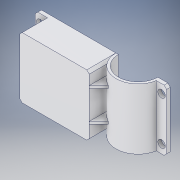
# Autodesk Inventor part: KS  Dianteiro Front
Saved by Autodesk Inventor 2019 (Build 230136000, 136)
## iProperties
Created: 2021-05-20
Part Number: KS  Dianteiro Front
Material: Genérico
Document SubType Name: Modeling
Designer: lukas
Density: 1 g/cm^3
Appearance: PTFE
Author: lukas
Autodesk Inventor part; units mm, degrees
ref_plane "YZ Plane" through (0, 0, 0) normal (1, 0, 0) x (0, 1, 0)
ref_plane "XZ Plane" through (0, 0, 0) normal (0, 1, 0) x (-1, 0, 0)
ref_plane "XY Plane" through (0, 0, 0) normal (0, 0, 1) x (1, 0, 0)
sketch "Esboço1" plane through (0, 0, 0) normal (0, 1, 0) x (-1, 0, 0)
  line L0 (-28, -11.75) -> (28, -11.75)
  line L1 (28, -11.75) -> (28, 11.75)
  line L2 (28, 11.75) -> (-28, 11.75)
  line L3 (-28, 11.75) -> (-28, -11.75)
  line L4 (-28, -11.75) -> (28, 11.75) construction
  line L5 (28, -11.75) -> (-28, 11.75) construction
  point P0 (0, 0)
  dimension "d0" = 56
  dimension "d1" = 23.5
  constraints: 12 end point, 2 midpoint, 2 parallel, 1 horizontal, 1 perpendicular
  measures "d0" distance of L2.end L1.end
  measures "d1" distance of L1.end L0.end
extrude "Extrusão1" add sketch "Esboço1" along normal blind 49
sketch "Esboço2" plane through (28, 0, -11.75) normal (0, 0, -1) x (-1, 0, 0)
  line L0 (0, 49) -> (56, 49) projected
  line L1 (0, 49) -> (-33.75, 49)
  line L2 (-33.75, 49) -> (-33.75, 0)
  line L3 (0, 0) -> (56, 0) projected
  line L4 (-33.75, 0) -> (0, 0)
  line L5 (0, 0) -> (0, 49)
  point P0 (28, 0)
  dimension "d4" = 33.75
  constraints: 8 end point, 3 perpendicular, 1 horizontal
  measures "d4" distance of L0.start L1.end
extrude "Extrusão2" add sketch "Esboço2" against normal blind 17.875
sketch "Esboço3" plane through (0, 49, 0) normal (0, 1, 0) x (1, 0, 0)
  line L0 (-28, 11.75) -> (61.75, 11.75) projected
  line L1 (61.75, 11.75) -> (59.75, 11.75)
  line L2 (59.75, 11.75) -> (43.875, 11.75)
  circle A0 centre (43.875, 11.75) radius 15.875
  point P0 (0, 0)
  dimension "d7" = 2
  dimension "d8" = 15.875
  constraints: 4 end point, 2 point on line, 1 coincident, 1 horizontal alignment, 2 other
  measures "d7" distance of L0.end L1.end
  measures "d8" distance of L1.end L2.end
extrude "Extrusão3" cut sketch "Esboço3" against normal blind 49
sketch "Esboço4" plane through (61.75, 0, -11.75) normal (0, 0, -1) x (-1, 0, 0)
  line L0 (0, 49) -> (33.75, 49) projected
  line L1 (33.75, 0) -> (0, 0) projected
  line L2 (0, 49) -> (0, 0)
  line L3 (0, 0) -> (-8, 0)
  line L4 (-8, 0) -> (-8, 49)
  line L5 (-8, 49) -> (0, 49)
  line L6 (-4, 0) -> (-4, 7)
  line L7 (-4, 49) -> (-4, 42)
  circle A0 centre (-4, 42) radius 3
  circle A1 centre (-4, 7) radius 3
  point P0 (61.75, 0)
  dimension "d11" = 8
  dimension "d12" = 7
  dimension "d13" = 7
  dimension "d14" = 6
  dimension "d15" = 6
  constraints: 12 end point, 3 vertical, 2 centre point, 2 coincident, 2 midpoint, 2 perpendicular, 1 horizontal
  measures "d11" distance of L1.end L3.end
  measures "d12" distance of L6.start L6.end
  measures "d13" distance of L7.start L7.end
  measures "d14" diameter of A0
  measures "d15" diameter of A1
extrude "Extrusão4" add sketch "Esboço4" against normal blind 3
sketch "Esboço5" plane through (0, 49, 0) normal (0, 1, 0) x (1, 0, 0)
  arc A0 (28, 11.75) -> (59.75, 11.75) centre (43.875, 11.75) ccw projected
  circle A1 centre (43.875, 11.75) radius 17.875
  line L0 (61.75, -6.125) -> (28, -6.125) projected
  line L1 (69.75, 8.75) -> (61.75, 8.75) projected
  line L2 (61.75, 8.75) -> (61.4965, 8.75)
  line L3 (61.75, 8.75) -> (61.75, -6.125)
  line L4 (43.875, -6.125) -> (61.75, -6.125)
  line L5 (28, -11.75) -> (28, -6.125) projected
  line L6 (43.875, -6.125) -> (28, -6.125)
  line L7 (28, -6.125) -> (28, 3.5342)
  point P0 (0, 0)
  constraints: 10 end point, 3 perpendicular, 3 point on circle, 2 tangent, 1 centre point, 1 coincident, 1 collinear, 1 horizontal, 1 point on line
extrude "Extrusão5" cut sketch "Esboço5" against normal blind 49 contours A1 L0 L7 | L2 L3 L0 A1
sketch "Esboço6" plane through (-28, 0, -11.75) normal (0, 0, -1) x (-1, 0, 0)
  line L0 (0, 0) -> (0, 49) projected
  line L1 (0, 49) -> (0, 0)
  line L2 (0, 0) -> (8, 0)
  line L3 (8, 0) -> (8, 49)
  line L4 (8, 49) -> (0, 49)
  line L5 (4, 49) -> (4, 42)
  line L6 (4, 0) -> (4, 7)
  circle A0 centre (4, 7) radius 3
  circle A1 centre (4, 42) radius 3
  point P0 (-28, 0)
  dimension "d20" = 8
  dimension "d21" = 7
  dimension "d22" = 7
  dimension "d23" = 6
  dimension "d24" = 6
  constraints: 12 end point, 3 perpendicular, 3 vertical, 2 centre point, 2 coincident, 2 midpoint
  measures "d20" distance of L0.start L2.end
  measures "d21" distance of L5.start L5.end
  measures "d22" distance of L6.start L6.end
  measures "d23" diameter of A0
  measures "d24" diameter of A1
extrude "Extrusão6" add sketch "Esboço6" against normal blind 3
sketch "Esboço8" plane through (28, 0, -11.75) normal (0, 0, -1) x (-1, 0, 0)
  line L0 (0, 49) -> (0, 0) projected
  line L1 (0, 49) -> (0, 47)
  line L2 (0, 47) -> (2, 47)
  line L3 (2, 47) -> (2, 2)
  line L4 (2, 47) -> (47, 47) construction
  line L5 (2, 2) -> (54, 2)
  line L6 (2, 2) -> (54, 2) construction
  line L7 (54, 2) -> (54, 47)
  line L8 (54, 47) -> (2, 47)
  point P0 (28, 0)
  dimension "d27" = 2
  dimension "d28" = 2
  dimension "d29" = 45
  dimension "d30" = 90
  dimension "d31" = 52
  dimension "d32" = 0
  constraints: 16 end point, 3 horizontal, 3 perpendicular, 2 equal length, 1 point on line, 1 vertical
  measures "d27" distance of L0.start L1.end
  measures "d28" distance of L1.end L2.end
  measures "d29" distance of L2.end L3.end
  measures "d30" angle of L3 L4
  measures "d31" distance of L3.end L5.end
  measures "d32" distance between parallel lines of L5 L6
extrude "Extrusão7" cut sketch "Esboço8" against normal blind 21.5
sketch "Esboço10" plane through (28, 0, 11.75) normal (1, 0, 0) x (0, 0, -1)
  line L0 (0, 0) -> (0, 49) projected
  line L1 (0, 49) -> (0, 37)
  line L2 (0, 0) -> (0, 12)
  line L3 (0, 12) -> (16, 12)
  line L4 (16, 12) -> (16, 14)
  line L5 (16, 14) -> (0, 14)
  line L6 (0, 12) -> (0, 14)
  line L7 (0, 37) -> (16, 37)
  line L8 (16, 37) -> (16, 39)
  line L9 (16, 39) -> (0, 39)
  point P0 (11.75, 0)
  dimension "d38" = 12
  dimension "d41" = 12
  dimension "d42" = 16
  dimension "d43" = 2
  dimension "d44" = 16
  dimension "d45" = 2
  constraints: 18 end point, 4 point on line, 2 horizontal, 2 perpendicular, 1 collinear, 1 parallel, 1 vertical
  measures "d38" distance of L0.end L1.end
  measures "d41" distance of L0.start L2.end
  measures "d42" distance of L2.end L3.end
  measures "d43" distance of L3.end L4.end
  measures "d44" distance of L1.end L7.end
  measures "d45" distance of L7.end L8.end
extrude "Extrusão9" add sketch "Esboço10" along normal blind 17.875
sketch "Esboço11" plane through (28, 39, 11.75) normal (0, 1, 0) x (1, 0, 0)
  arc A0 (0, 15.2842) -> (33.4965, 20.5) centre (15.875, 23.5) ccw projected
  arc A1 (0, 23.5) -> (31.75, 23.5) centre (15.875, 23.5) ccw projected
  line L0 (17.875, 0) -> (17.875, 5.7372) projected
  line L1 (17.875, 5.7372) -> (17.875, 0)
  line L2 (0, 0) -> (17.875, 0) projected
  line L3 (17.875, 0) -> (0, 0)
  line L4 (0, 0) -> (7.6367, 7.6367)
  arc A2 (0, 15.2842) -> (17.875, 5.7372) centre (15.875, 23.5) ccw projected
  arc A3 (7.6367, 7.6367) -> (17.875, 5.7372) centre (15.875, 23.5) ccw
  line L5 (1.8834, 16) -> (17.875, 16) projected
  line L6 (1.8834, 16) -> (17.875, 16)
  line L7 (17.875, 16) -> (17.875, 7.7515) projected
  line L8 (17.875, 16) -> (17.875, 7.7515)
  arc A4 (1.8834, 16) -> (17.875, 7.7515) centre (15.875, 23.5) ccw
  point P0 (-28, 11.75)
  dimension "d48" = 45
  constraints: 10 end point, 5 point on circle, 4 collinear, 2 centre point, 2 coincident
  measures "d48" angle of L3 L4
extrude "Extrusão10" cut sketch "Esboço11" against normal blind 27.875
chamfer "Chanfro1" distance 2 angle 45 8 edges at (28, 49, 4.1079) (28, 0, 4.1079) (-28, 0, 1.5) (-28, 49, 1.5) (69.75, 49, -10.25) (69.75, 0, -10.25) (-36, 49, -10.25) (-36, 0, -10.25)
